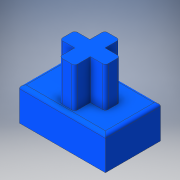
# Autodesk Inventor part: keyswitch-pole_cherrymx
Saved by Autodesk Inventor 2016 (Build 200138000, 138)
## iProperties
Created: 2016-12-08
Part Number: keyswitch-pole_cherrymx
Material: Generic
Document SubType Name: Modeling
Designer: Cemra JC
Density: 1 g/cm^3
Appearance: Default
Author: Cemra JC
Autodesk Inventor part; units mm, degrees
ref_plane "YZ Plane" through (0, 0, 0) normal (1, 0, 0) x (0, 1, 0)
ref_plane "XZ Plane" through (0, 0, 0) normal (0, 1, 0) x (-1, 0, 0)
ref_plane "XY Plane" through (0, 0, 0) normal (0, 0, 1) x (1, 0, 0)
sketch "Sketch1" plane through (0, 0, 0) normal (0, 1, 0) x (-1, 0, 0)
  line L0 (3.9, 2.5) -> (-3.9, 2.5)
  line L1 (-3.9, 2.5) -> (-3.9, -2.5)
  line L2 (-3.9, -2.5) -> (3.9, -2.5)
  line L3 (3.9, -2.5) -> (3.9, 2.5)
  line L4 (3.9, 2.5) -> (-3.9, -2.5) construction
  line L5 (-3.9, 2.5) -> (3.9, -2.5) construction
  point P0 (0, 0)
  dimension "d0" = 7.8
  dimension "d1" = 5
  constraints: 12 end point, 2 midpoint, 2 parallel, 1 horizontal, 1 perpendicular
  measures "d0" distance of L1.end L2.end
  measures "d1" distance of L2.end L0.start
extrude "Pole Base" add sketch "Sketch1" along normal blind 3
sketch "Sketch2" plane through (0, 3, 0) normal (0, 1, 0) x (1, 0, 0)
  line L0 (0.7, -2.0872) -> (-0.7, -2.0872)
  line L1 (-0.675, 2.0127) -> (0.675, 2.0127)
  line L2 (0.7, -2.0872) -> (-0.675, 2.0127) construction
  line L3 (-0.7, -2.0872) -> (0.675, 2.0127) construction
  line L4 (-2.05, -0.6873) -> (-2.05, 0.6627)
  line L5 (2.05, 0.6873) -> (2.05, -0.6627)
  line L6 (2.05, -0.6627) -> (-2.05, 0.6627) construction
  line L7 (-2.05, -0.6873) -> (2.05, 0.6873) construction
  line L8 (2.05, -0.6627) -> (0.7, -0.6627)
  line L9 (-0.7, -0.6873) -> (-2.05, -0.6873)
  line L10 (-0.7, -2.0872) -> (-0.7, -0.6873)
  line L11 (-0.675, 0.6627) -> (-0.675, 2.0127)
  line L12 (-2.05, 0.6627) -> (-0.675, 0.6627)
  line L13 (0.675, 0.6873) -> (2.05, 0.6873)
  line L14 (0.675, 2.0127) -> (0.675, 0.6873)
  line L15 (0.7, -0.6627) -> (0.7, -2.0872)
  point P0 (0, 0)
  dimension "d4" = 1.35
  dimension "d5" = 4.1
  dimension "d6" = 4.1
  dimension "d7" = 1.35
  constraints: 32 end point, 10 parallel, 8 perpendicular, 3 horizontal, 2 midpoint, 2 point on line
  measures "d4" distance of L1.start L1.end
  measures "d5" distance of L0.end L1.start
  measures "d6" distance of L4.end L5.start
  measures "d7" distance of L4.start L4.end
extrude "Pole" add sketch "Sketch2" along normal blind 3.6
fillet "Pole Rounding" radius 0.25 8 edges at (0.7, 4.8, 2.0872) (2.05, 4.8, 0.6627) (-0.7, 4.8, 2.0872) (2.05, 4.8, -0.6873) (0.675, 4.8, -2.0127) (-0.675, 4.8, -2.0127) (-2.05, 4.8, -0.6627) (-2.05, 4.8, 0.6873)
fillet "Base Rounding" radius 0.3 4 edges at (-3.9, 3, 0) (0, 3, -2.5) (0, 3, 2.5) (3.9, 3, 0)
body "Solid1"
